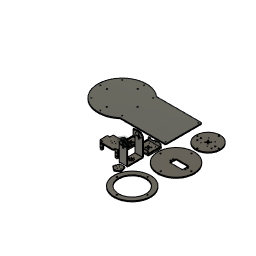
Adaptive Robot (Autodesk Fusion 360 design; units mm, degrees)
Autodesk Fusion 360 part; units mm, degrees
(part 1 of 2)
sketch "Sketch1" plane through (0, 0, 0) normal (0, 0, 1) x (1, 0, 0) in component "Base Plate"
  circle A0 centre (0, 0) radius 80
  line L0 (52.915, 60) -> (52.915, -60)
  line L1 (52.915, -60) -> (199.915, -60)
  line L2 (202.915, -57) -> (202.915, 57)
  line L3 (199.915, 60) -> (52.915, 60)
  line L4 (202.915, 0) -> (52.915, 0) construction
  arc A1 (202.915, 57) -> (199.915, 60) centre (199.915, 57) ccw
  arc A2 (199.915, -60) -> (202.915, -57) centre (199.915, -57) ccw
  circle A3 centre (0, 72) radius 1.5
  line L5 (0, 0) -> (0, 80) construction
  circle A4 centre (-50.9117, 50.9117) radius 1.5
  circle A5 centre (-72, 0) radius 1.5
  circle A6 centre (-50.9117, -50.9117) radius 1.5
  circle A7 centre (0, -72) radius 1.5
  circle A8 centre (50.9117, -50.9117) radius 1.5
  circle A9 centre (50.9117, 50.9117) radius 1.5
  line L6 (-50.9117, 50.9117) -> (50.9117, 50.9117) construction
  line L7 (-50.9117, -50.9117) -> (-50.9117, 50.9117) construction
  circle A10 centre (0, 50.9117) radius 2
  circle A11 centre (-50.9117, 0) radius 2
  circle A12 centre (0, -50.9117) radius 2
  circle A13 centre (50.9117, 0) radius 2
  circle A14 centre (196.915, 54) radius 1.5
  circle A15 centre (196.915, -54) radius 1.5
  point P0 (202.915, 60)
  dimension "d2" = 120
  dimension "d3" = 160
  dimension "d4" = 150
  dimension "d5" = 3
  dimension "d6" = 3
  dimension "d8" = 8
  dimension "d10" = 360
  dimension "d13" = 4
  dimension "d15" = 360
  dimension "d20" = 3
  dimension "d21" = 6
  dimension "d22" = 6
  dimension "d23" = 3
  dimension "d24" = 6
  dimension "d25" = 6
  constraint coincident A0.centre L5.start
  constraint perpendicular L0 L1
  constraint parallel L0 L2
  constraint parallel L1 L3
  constraint coincident A0 L0.end
  constraint vertical L0
  constraint coincident A0 L0.start
  constraint midpoint L0 L4.end
  constraint coincident L2 L4.start
  constraint coincident P0 L2
  constraint coincident P0 L3
  constraint tangent L2 A1
  constraint tangent L3 A1
  constraint tangent L1 A2
  constraint tangent L2 A2
  constraint equal A1 A2
  constraint coincident A0 L5.end
  constraint vertical L5
  constraint coincident A3.centre L5
  constraint coincident A4.centre L6.start
  constraint coincident A9.centre L6.end
  constraint coincident A6.centre L7.start
  constraint midpoint L6 A10.centre
  measures "d2" distance of L1 L3
  measures "d3" diameter of A0
  measures "d4" distance of L0.start P0
  measures "d5" radius of A1
  measures "d6" diameter of A3
  measures "d8" distance of A3.centre L5.end
  measures "d13" diameter of A10
  measures "d20" diameter of A14
  measures "d21" distance of L3 A14.centre
  measures "d22" distance of L2 A14.centre
  measures "d23" diameter of A15
  measures "d24" distance of L1 A15.centre
  measures "d25" distance of L2 A15.centre
extrude "Extrude3" add sketch "Sketch1" along normal blind 3 contours A0 L0 | A0 L1 L2 L3 A1 A2 | A0 L0 | A14 | A15 makes body 1 in component "Base Plate"
extrude "Extrude4" cut sketch "Sketch1" along normal blind 3 contours A14 | A15 bodies 1 in component "Base Plate"
sketch "Sketch1 (2)" plane through (0, 0, 0) normal (0, 0, 1) x (1, 0, 0) in component "CircularL"
  circle A0 centre (131.6018, -175.8664) radius 40
  circle A1 centre (131.6018, -175.8664) radius 4
  circle A2 centre (131.6018, -140.3664) radius 2
  line L0 (131.6018, -175.8664) -> (131.6018, -135.8664) construction
  circle A3 centre (96.1018, -175.8664) radius 2
  circle A4 centre (131.6018, -211.3664) radius 2
  circle A5 centre (167.1018, -175.8664) radius 2
  line L1 (96.1018, -175.8664) -> (167.1018, -175.8664) construction
  circle A6 centre (108.1018, -175.8664) radius 2
  line L2 (108.1018, -175.8664) -> (108.1018, -208.2353) construction
  circle A7 centre (108.1018, -187.8664) radius 2
  circle A8 centre (155.1018, -187.8664) radius 2
  circle A9 centre (155.1018, -175.8664) radius 2
  line L3 (131.6018, -175.8664) -> (159.8861, -147.5821) construction
  circle A10 centre (136.5516, -170.9166) radius 1.5
  circle A11 centre (126.6521, -170.9166) radius 1.5
  circle A12 centre (126.6521, -180.8161) radius 1.5
  circle A13 centre (136.5516, -180.8161) radius 1.5
  line L4 (131.6018, -162.3664) -> (93.9488, -162.3664) construction
  dimension "d30" = 80
  dimension "d31" = 8
  dimension "d32" = 4
  dimension "d33" = 4.5
  dimension "d35" = 360
  dimension "d36" = 4
  dimension "d37" = 12
  dimension "d38" = 4
  dimension "d39" = 12
  dimension "d40" = 45
  dimension "d41" = 3
  dimension "d42" = 7
  dimension "d44" = 360
  dimension "d46" = 13.5
  constraint concentric A0 A1
  constraint coincident A0.centre A1.centre
  constraint coincident A0 L0.end
  constraint vertical L0
  constraint coincident A2.centre L0
  constraint coincident A3.centre L1.start
  constraint coincident A5.centre L1.end
  constraint coincident L1 A6.centre
  constraint coincident A6.centre L2.start
  constraint perpendicular L1 L2
  constraint coincident L2 A7.centre
  constraint coincident A0 L2.end
  constraint symmetric L0 A6 A9
  constraint symmetric L0 A7 A8
  constraint coincident A0 L3.end
  constraint coincident L3 A10.centre
  constraint coincident A0 L4.end
  constraint perpendicular L0 L4
  measures "d30" diameter of A0
  measures "d31" diameter of A1
  measures "d32" diameter of A2
  measures "d33" distance of A2.centre L0.end
  measures "d36" diameter of A6
  measures "d37" distance of A3.centre A6.centre
  measures "d38" diameter of A7
  measures "d39" distance of A6.centre A7.centre
  measures "d40" angle of L1 L3
  measures "d41" diameter of A10
  measures "d42" distance of A0.centre A10.centre
  measures "d46" distance of A0.centre L4.start
extrude "Extrude1" add sketch "Sketch1 (2)" along normal blind 3 separate body makes body 2 in component "CircularL"
sketch "Sketch1 (3)" plane through (0, 0, 0) normal (0, 0, 1) x (1, 0, 0) in component "ServoHolder"
  line L0 (60.9854, -112.0365) -> (103.9854, -112.0365)
  line L1 (103.9854, -112.0365) -> (103.9854, -155.0365)
  line L2 (103.9854, -155.0365) -> (60.9854, -155.0365)
  line L3 (60.9854, -155.0365) -> (60.9854, -112.0365)
  line L4 (82.4854, -112.0365) -> (82.4854, -155.0365) construction
  line L5 (60.9854, -133.5365) -> (103.9854, -133.5365) construction
  circle A0 centre (82.4854, -133.5365) radius 4
  circle A1 centre (95.9854, -123.0365) radius 1
  line L6 (95.9854, -123.0365) -> (95.9854, -155.0365) construction
  circle A2 centre (95.9854, -144.0365) radius 1
  circle A3 centre (68.9854, -144.0365) radius 1
  circle A4 centre (68.9854, -123.0365) radius 1
  dimension "d51" = 43
  dimension "d52" = 43
  dimension "d53" = 8
  dimension "d54" = 2
  dimension "d55" = 11
  dimension "d56" = 8
  constraint horizontal L0
  constraint vertical L1
  constraint horizontal L2
  constraint vertical L3
  constraint midpoint L0 L4.start
  constraint midpoint L2 L4.end
  constraint midpoint L3 L5.start
  constraint midpoint L1 L5.end
  constraint midpoint L5 A0.centre
  constraint coincident A1.centre L6.start
  constraint coincident L2 L6.end
  constraint perpendicular L2 L6
  constraint symmetric L5 A1 A2
  constraint symmetric L4 A1 A4
  constraint symmetric L4 A2 A3
  measures "d51" distance of L1 L3
  measures "d52" distance of L0 L2
  measures "d53" diameter of A0
  measures "d54" diameter of A1
  measures "d55" distance of L0 A1.centre
  measures "d56" distance of L1 A1.centre
extrude "Extrude1'" add sketch "Sketch1 (3)" along normal blind 3 separate body makes body 3 in component "ServoHolder"
sketch "Sketch2" plane through (0, 0, 3) normal (0, 0, 1) x (-1, 0, 0) in component "ServoHolder"
  circle A0 centre (-95.9854, 123.0365) radius 1
  circle A1 centre (-95.9854, 144.0365) radius 1
  circle A2 centre (-68.9854, 123.0365) radius 1
  circle A3 centre (-82.4854, 133.5365) radius 4
  circle A4 centre (-68.9854, 144.0365) radius 1
  line L0 (-60.9854, 155.0365) -> (-103.9854, 155.0365)
  line L1 (-103.9854, 155.0365) -> (-103.9854, 112.0365)
  line L2 (-103.9854, 112.0365) -> (-60.9854, 112.0365)
  line L3 (-60.9854, 112.0365) -> (-60.9854, 155.0365)
  line L4 (-60.9854, 112.0365) -> (-103.9854, 112.0365)
  line L5 (-103.9854, 112.0365) -> (-103.9854, 113.0365)
  line L6 (-103.9854, 113.0365) -> (-60.9854, 113.0365)
  line L7 (-60.9854, 113.0365) -> (-60.9854, 112.0365)
  line L8 (-60.9854, 155.0365) -> (-103.9854, 155.0365)
  line L9 (-103.9854, 155.0365) -> (-103.9854, 154.0365)
  line L10 (-103.9854, 154.0365) -> (-60.9854, 154.0365)
  line L11 (-60.9854, 154.0365) -> (-60.9854, 155.0365)
  dimension "d59" = 1
  dimension "d60" = 1
  constraint horizontal L4
  constraint vertical L5
  constraint horizontal L6
  constraint vertical L7
  constraint coincident L1 L5.end
  constraint coincident L2.end L3.start
  constraint horizontal L8
  constraint vertical L9
  constraint horizontal L10
  constraint vertical L11
  constraint coincident L1 L9.end
  constraint coincident L0.start L3.end
  measures "d59" distance of L0.end L9.end
  measures "d60" distance of L1.end L5.end
extrude "Extrude2" add sketch "Sketch2" along normal blind 3 contours L0 L1 L3 L8 L9 L10 L11 | L1 L2 L3 L4 L5 L6 L7 bodies 3 in component "ServoHolder"
sketch "Sketch3" plane through (0, 0, 3) normal (0, 0, 1) x (-1, 0, 0) in component "ServoHolder"
  line L0 (-60.9854, 154.0365) -> (-103.9854, 154.0365)
  line L1 (-103.9854, 154.0365) -> (-103.9854, 113.0365)
  line L2 (-103.9854, 113.0365) -> (-60.9854, 113.0365)
  line L3 (-60.9854, 113.0365) -> (-60.9854, 154.0365)
  circle A0 centre (-68.9854, 144.0365) radius 1
  circle A1 centre (-82.4854, 133.5365) radius 4
  circle A2 centre (-68.9854, 123.0365) radius 1
  circle A3 centre (-95.9854, 144.0365) radius 1
  circle A4 centre (-95.9854, 123.0365) radius 1
  line L4 (-60.9854, 113.0365) -> (-61.9854, 113.0365)
  line L5 (-61.9854, 113.0365) -> (-61.9854, 154.0365)
  line L6 (-61.9854, 154.0365) -> (-60.9854, 154.0365)
  line L7 (-60.9854, 154.0365) -> (-60.9854, 113.0365)
  line L8 (-103.9854, 113.0365) -> (-102.9854, 113.0365)
  line L9 (-102.9854, 113.0365) -> (-102.9854, 154.0365)
  line L10 (-102.9854, 154.0365) -> (-103.9854, 154.0365)
  line L11 (-103.9854, 154.0365) -> (-103.9854, 113.0365)
  dimension "d63" = 1
  dimension "d64" = 1
  constraint horizontal L4
  constraint vertical L5
  constraint horizontal L6
  constraint vertical L7
  constraint coincident L0 L5.end
  constraint coincident L2.end L3.start
  constraint horizontal L8
  constraint vertical L9
  constraint horizontal L10
  constraint vertical L11
  constraint coincident L0 L9.end
  constraint coincident L1.end L2.start
  measures "d63" distance of L2.end L4.end
  measures "d64" distance of L1.end L8.end
extrude "Extrude3'" add sketch "Sketch3" along normal blind 10 contours L0 L2 L3 L4 L5 L6 L7 | L0 L1 L2 L8 L9 L10 L11 bodies 3 in component "ServoHolder"
sketch "Sketch4" plane through (60.9854, 0, 0) normal (-1, 0, 0) x (0, -1, 0) in component "ServoHolder"
  line L0 (112.0365, 0) -> (155.0365, 0)
  line L1 (155.0365, 0) -> (155.0365, 6)
  line L2 (155.0365, 6) -> (154.0365, 6)
  line L3 (154.0365, 6) -> (154.0365, 13)
  line L4 (154.0365, 13) -> (113.0365, 13)
  line L5 (113.0365, 13) -> (113.0365, 6)
  line L6 (113.0365, 6) -> (112.0365, 6)
  line L7 (112.0365, 6) -> (112.0365, 0)
  line L8 (134.0365, 13) -> (137.5365, 9)
  line L9 (137.5365, 9) -> (141.5365, 9)
  line L10 (141.5365, 9) -> (141.5365, 13)
  line L11 (149.0365, 13) -> (145.5365, 9)
  line L12 (145.5365, 9) -> (141.5365, 9)
  dimension "d67" = 4
  dimension "d68" = 4
  dimension "d69" = 3.5
  dimension "d70" = 21
  constraint coincident L4 L8.start
  constraint horizontal L9
  constraint coincident L4 L10.end
  constraint perpendicular L4 L10
  constraint symmetric L8.start L10 L11.start
  constraint symmetric L8.end L10 L11.end
  constraint symmetric L9.end L10 L12.end
  measures "d67" distance of L8.end L9.end
  measures "d68" distance of L9.end L10.end
  measures "d69" horizontal distance of L8.start L8.end
  measures "d70" distance of L4.end L8.start
extrude "Extrude4'" cut sketch "Sketch4" against normal blind 43 contours L4 L8 L9 L10 | L4 L10 L11 L12 bodies 3 in component "ServoHolder"
sketch "Sketch5" plane through (60.9854, 0, 0) normal (-1, 0, 0) x (0, -1, 0) in component "ServoHolder"
  line L0 (149.0365, 13) -> (145.5365, 9)
  line L1 (145.5365, 9) -> (137.5365, 9)
  line L2 (137.5365, 9) -> (134.0365, 13)
  line L3 (134.0365, 13) -> (113.0365, 13)
  line L4 (113.0365, 13) -> (113.0365, 6)
  line L5 (113.0365, 6) -> (112.0365, 6)
  line L6 (112.0365, 6) -> (112.0365, 0)
  line L7 (112.0365, 0) -> (155.0365, 0)
  line L8 (155.0365, 0) -> (155.0365, 6)
  line L9 (155.0365, 6) -> (154.0365, 6)
  line L10 (154.0365, 6) -> (154.0365, 13)
  line L11 (154.0365, 13) -> (149.0365, 13)
  circle A0 centre (115.5365, 9) radius 1
  circle A1 centre (130.5365, 9) radius 1
  circle A2 centre (151.5365, 9) radius 1
  line L12 (113.0365, 9) -> (154.0365, 9) construction
  dimension "d73" = 2
  dimension "d74" = 2
  dimension "d75" = 2
  dimension "d76" = 4
  dimension "d77" = 2.5
  dimension "d78" = 2.5
  dimension "d79" = 15
  constraint coincident L4 L12.start
  constraint coincident L10 L12.end
  constraint perpendicular L10 L12
  constraint coincident A0.centre L12
  constraint coincident A1.centre L12
  constraint coincident A2.centre L12
  measures "d73" diameter of A0
  measures "d74" diameter of A1
  measures "d75" diameter of A2
  measures "d76" distance of L3 L12
  measures "d77" distance of A2.centre L12.end
  measures "d78" distance of A0.centre L12.start
  measures "d79" distance of A0.centre A1.centre
extrude "Extrude5" cut sketch "Sketch5" against normal blind 43 contours A0 | A1 | A2 bodies 3 in component "ServoHolder"
sketch "Sketch3 (2)" plane through (0, 0, 3) normal (0, 0, 1) x (-1, 0, 0) in component "CircularL"
  circle A0 centre (-136.5516, 170.9166) radius 1.5
  circle A1 centre (-155.1018, 175.8664) radius 2
  circle A2 centre (-155.1018, 187.8664) radius 2
  circle A3 centre (-108.1018, 187.8664) radius 2
  circle A4 centre (-108.1018, 175.8664) radius 2
  circle A5 centre (-167.1018, 175.8664) radius 2
  circle A6 centre (-131.6018, 211.3664) radius 2
  circle A7 centre (-96.1018, 175.8664) radius 2
  circle A8 centre (-131.6018, 140.3664) radius 2
  circle A9 centre (-131.6018, 175.8664) radius 4
  circle A10 centre (-126.6521, 170.9166) radius 1.5
  circle A11 centre (-126.6521, 180.8161) radius 1.5
  circle A12 centre (-136.5516, 180.8161) radius 1.5
  circle A13 centre (-131.6018, 175.8664) radius 40
  circle A14 centre (-359.9097, 287.882) radius 1
  circle A15 centre (-359.9097, 266.882) radius 1
  circle A16 centre (-386.9097, 266.882) radius 1
  circle A17 centre (-386.9097, 287.882) radius 1
extrude "Extrude2'" cut sketch "Sketch3 (2)" against normal blind 3 contours A14 | A15 | A16 | A17 bodies 2 in component "CircularL"
sketch "Sketch6" plane through (0, 0, 3) normal (0, 0, 1) x (-1, 0, 0) in component "ServoHolder"
  line L0 (-102.9854, 154.0365) -> (-102.9854, 113.0365)
  line L1 (-102.9854, 113.0365) -> (-61.9854, 113.0365)
  line L2 (-61.9854, 113.0365) -> (-61.9854, 154.0365)
  line L3 (-61.9854, 154.0365) -> (-102.9854, 154.0365)
  circle A0 centre (-68.9854, 144.0365) radius 1
  circle A1 centre (-82.4854, 133.5365) radius 4
  circle A2 centre (-68.9854, 123.0365) radius 1
  circle A3 centre (-95.9854, 144.0365) radius 1
  circle A4 centre (-95.9854, 123.0365) radius 1
  circle A5 centre (154.3727, 27.0711) radius 1.5
  circle A6 centre (164.2722, 27.0711) radius 1.5
  circle A7 centre (164.2722, 36.9706) radius 1.5
  circle A8 centre (154.3727, 36.9706) radius 1.5
  circle A9 centre (154.3727, 27.0711) radius 1
  circle A10 centre (154.3727, 36.9706) radius 1
  circle A11 centre (164.2722, 27.0711) radius 1
  circle A12 centre (164.2722, 36.9706) radius 1
  dimension "d102" = 2
  dimension "d103" = 2
  dimension "d104" = 2
  dimension "d105" = 2
  constraint concentric A5 A9
  constraint concentric A8 A10
  constraint concentric A6 A11
  constraint concentric A7 A12
  measures "d102" diameter of A9
  measures "d103" diameter of A10
  measures "d104" diameter of A11
  measures "d105" diameter of A12
extrude "Extrude6" cut sketch "Sketch6" against normal blind 3 contours A9 | A10 | A11 | A12 bodies 3 in component "ServoHolder"
sketch "Sketch1 (4)" plane through (0, 0, 0) normal (0, 0, 1) x (1, 0, 0) in component "ServoCutOut"
  circle A0 centre (-2.8865, -157.1678) radius 60
  dimension "d108" = 120
  measures "d108" diameter of A0
extrude "Extrude1''" add sketch "Sketch1 (4)" along normal blind 3 separate body makes body 4 in component "ServoCutOut"
sketch "Sketch2 (2)" plane through (0, 0, 3) normal (0, 0, 1) x (-1, 0, 0) in component "ServoCutOut"
  circle A0 centre (2.8865, 157.1678) radius 60
  circle A1 centre (-196.915, -54) radius 1.5
  circle A2 centre (-196.915, 54) radius 1.5
  circle A3 centre (0, -50.9117) radius 2
  circle A4 centre (-50.9117, -50.9117) radius 1.5
  circle A5 centre (-50.9117, 50.9117) radius 1.5
  circle A6 centre (0, 72) radius 1.5
  circle A7 centre (72, 0) radius 1.5
  circle A8 centre (50.9117, -50.9117) radius 1.5
  circle A9 centre (0, -72) radius 1.5
  circle A10 centre (50.9117, 50.9117) radius 1.5
  circle A11 centre (0, 50.9117) radius 2
  circle A12 centre (50.9117, 0) radius 2
  circle A13 centre (-50.9117, 0) radius 2
  arc A14 (-199.915, 60) -> (-202.915, 57) centre (-199.915, 57) ccw
  line L0 (-199.915, 60) -> (-52.915, 60)
  arc A15 (-52.915, -60) -> (-52.915, 60) centre (0, 0) ccw
  line L1 (-52.915, -60) -> (-199.915, -60)
  arc A16 (-202.915, -57) -> (-199.915, -60) centre (-199.915, -57) ccw
  line L2 (-202.915, -57) -> (-202.915, 57)
extrude "Extrude2''" cut sketch "Sketch2 (2)" against normal blind 3 contours A3 | A11 | A12 | A13 bodies 4 in component "ServoCutOut"
sketch "Sketch3 (3)" plane through (0, 0, 3) normal (0, 0, 1) x (-1, 0, 0) in component "ServoCutOut"
  circle A0 centre (2.8865, 157.1678) radius 60
  line L0 (2.8865, 157.1678) -> (4.4061, 157.1678)
  line L1 (4.4061, 157.1678) -> (62.8865, 157.1678) construction
  line L2 (2.8865, 157.1678) -> (-57.1135, 157.1678) construction
  line L3 (2.8865, 157.1678) -> (2.8865, 155.2869)
  line L4 (2.8865, 155.2869) -> (2.8865, 97.1678) construction
  line L5 (2.8865, 157.1678) -> (2.8865, 217.1678) construction
  line L6 (-28.1135, 167.6678) -> (12.8865, 167.6678)
  line L7 (12.8865, 167.6678) -> (12.8865, 146.6678)
  line L8 (12.8865, 146.6678) -> (-28.1135, 146.6678)
  line L9 (-28.1135, 146.6678) -> (-28.1135, 167.6678)
  line L10 (-28.1135, 167.6678) -> (12.8865, 146.6678) construction
  line L11 (12.8865, 167.6678) -> (-28.1135, 146.6678) construction
  circle A1 centre (12.8865, 157.1678) radius 1.5
  circle A2 centre (-28.1135, 157.1678) radius 1.5
  circle A3 centre (16.8865, 153.1678) radius 2
  circle A4 centre (16.8865, 161.1678) radius 2
  line L12 (-7.6135, 157.1678) -> (-7.6135, 146.6678) construction
  circle A5 centre (-32.1135, 153.1678) radius 2
  circle A6 centre (-32.1135, 161.1678) radius 2
  point P0 (-7.6135, 157.1678)
  point P1 (12.8865, 157.1678)
  dimension "d117" = 41
  dimension "d118" = 21
  dimension "d119" = 10
  dimension "d120" = 3
  dimension "d121" = 3
  dimension "d124" = 4
  dimension "d125" = 4
  dimension "d126" = 4
  constraint coincident A0.centre L0.start
  constraint horizontal L0
  constraint coincident A0 L1.end
  constraint parallel L0 L1
  constraint coincident A0 L2.end
  constraint parallel L0 L2
  constraint perpendicular L0 L3
  constraint coincident A0 L4.end
  constraint perpendicular L0 L4
  constraint coincident A0 L5.end
  constraint perpendicular L1 L5
  constraint horizontal L6
  constraint perpendicular L6 L7
  constraint parallel L6 L8
  constraint parallel L7 L9
  constraint coincident L10 P0
  constraint coincident L11 P0
  constraint coincident L2 P0
  constraint midpoint L7 P1
  constraint coincident P1 A1.centre
  constraint midpoint L9 A2.centre
  constraint symmetric L1 A3 A4
  constraint coincident P0 L12.start
  constraint midpoint L8 L12.end
  constraint symmetric A3 L12 A5
  constraint symmetric A4 L12 A6
  measures "d117" distance of L6.start L6.end
  measures "d118" distance of L6.start L8.end
  measures "d119" distance of A0.centre P1
  measures "d120" diameter of A1
  measures "d121" diameter of A2
  measures "d124" diameter of A3
  measures "d125" distance of L7 A3.centre
  measures "d126" distance of L1 A3.centre
extrude "Extrude4''" cut sketch "Sketch3 (3)" against normal blind 3 contours A3 | A4 | A5 | A6 bodies 4 in component "ServoCutOut"
extrude "Extrude3''" cut sketch "Sketch3 (3)" against normal blind 3 contours L6 L7 L8 L9 A1 A2 | L9 A2 | L9 A2 | L7 A1 | L7 A1 bodies 4 in component "ServoCutOut"
sketch "Sketch1 (5)" plane through (-2.8865, -157.1678, 3) normal (0, 0, 1) x (-1, 0, 0) in component "BearingOutside"
  line L0 (10, 10.5) -> (10, 1.5)
  arc A0 (10, -1.5) -> (10, 1.5) centre (10, 0) ccw
  line L1 (10, -1.5) -> (10, -10.5)
  line L2 (10, -10.5) -> (-31, -10.5)
  line L3 (-31, -10.5) -> (-31, -1.5)
  arc A1 (-31, 1.5) -> (-31, -1.5) centre (-31, 0) ccw
  line L4 (-31, 1.5) -> (-31, 10.5)
  line L5 (-31, 10.5) -> (10, 10.5)
  circle A2 centre (14, 4) radius 2
  circle A3 centre (-35, -4) radius 2
  circle A4 centre (14, -4) radius 2
  circle A5 centre (-35, 4) radius 2
  circle A6 centre (0, 0) radius 60
  circle A7 centre (0, 0) radius 60
  circle A8 centre (0, 0) radius 45
  dimension "d129" = 90
  constraint concentric A6 A7
  constraint concentric A7 A8
  measures "d129" diameter of A8
extrude "Extrude1'''" add sketch "Sketch1 (5)" along normal blind 3 separate body contours A6 A7 makes body 5 in component "BearingOutside"
sketch "Sketch1 (6)" plane through (0, 0, 0) normal (0, 0, 1) x (1, 0, 0) in component "UConnector"
  line L0 (-1.0772, -105.7415) -> (23.9228, -105.7415)
  line L1 (23.9228, -105.7415) -> (23.9228, -160.7415)
  line L2 (23.9228, -160.7415) -> (-1.0772, -160.7415)
  line L3 (-1.0772, -160.7415) -> (-1.0772, -105.7415)
  dimension "d132" = 25
  dimension "d133" = 55
  constraint horizontal L0
  constraint vertical L1
  constraint horizontal L2
  constraint vertical L3
  measures "d132" distance of L0.start L0.end
  measures "d133" distance of L0.end L1.end
extrude "Extrude1''''" add sketch "Sketch1 (6)" along normal blind 3 separate body makes body 6 in component "UConnector"
sketch "Sketch2 (3)" plane through (0, 0, 3) normal (0, 0, 1) x (-1, 0, 0) in component "UConnector"
  line L0 (1.0772, 160.7415) -> (-23.9228, 160.7415)
  line L1 (-23.9228, 160.7415) -> (-23.9228, 105.7415)
  line L2 (-23.9228, 105.7415) -> (1.0772, 105.7415)
  line L3 (1.0772, 105.7415) -> (1.0772, 160.7415)
  line L4 (1.0772, 105.7415) -> (-23.9228, 105.7415)
  line L5 (-23.9228, 105.7415) -> (-23.9228, 108.7415)
  line L6 (-23.9228, 108.7415) -> (1.0772, 108.7415)
  line L7 (1.0772, 108.7415) -> (1.0772, 105.7415)
  line L8 (1.0772, 160.7415) -> (-23.9228, 160.7415)
  line L9 (-23.9228, 160.7415) -> (-23.9228, 157.7415)
  line L10 (-23.9228, 157.7415) -> (1.0772, 157.7415)
  line L11 (1.0772, 157.7415) -> (1.0772, 160.7415)
  dimension "d136" = 3
  dimension "d137" = 3
  constraint horizontal L4
  constraint vertical L5
  constraint horizontal L6
  constraint vertical L7
  constraint coincident L1 L5.end
  constraint coincident L2.end L3.start
  constraint horizontal L8
  constraint vertical L9
  constraint horizontal L10
  constraint vertical L11
  constraint coincident L1 L9.end
  constraint coincident L0.start L3.end
  measures "d136" distance of L0.end L9.end
  measures "d137" distance of L1.end L5.end
extrude "Extrude2'''" add sketch "Sketch2 (3)" along normal blind 65 contours L0 L1 L3 L8 L9 L10 L11 | L1 L2 L3 L4 L5 L6 L7 bodies 6 in component "UConnector"
fillet "Fillet1" radius 12.5 4 edges at (-1.0772, -107.2415, 68) (23.9228, -107.2415, 68) (23.9228, -159.2415, 68) (-1.0772, -159.2415, 68) on bodies 6 in component "UConnector"
sketch "Sketch3 (4)" plane through (0, -160.7415, 0) normal (0, -1, 0) x (1, 0, 0) in component "UConnector"
  arc A0 (23.9228, 55.5) -> (-1.0772, 55.5) centre (11.4228, 55.5) ccw
  line L0 (-1.0772, 55.5) -> (-1.0772, 0)
  line L1 (-1.0772, 0) -> (23.9228, 0)
  line L2 (23.9228, 0) -> (23.9228, 55.5)
  line L3 (-1.0772, 55.5) -> (23.9228, 55.5) construction
  circle A1 centre (11.4228, 55.5) radius 4
  circle A2 centre (4.4228, 55.5) radius 1.5
  circle A3 centre (11.4228, 48.5) radius 1.5
  circle A4 centre (18.4228, 55.5) radius 1.5
  circle A5 centre (11.4228, 62.5) radius 1.5
  dimension "d142" = 8
  dimension "d143" = 3
  dimension "d144" = 7
  dimension "d146" = 360
  constraint coincident A0.end L0.start
  constraint coincident A0.start L2.end
  constraint concentric A0 A1
  constraint coincident L3 A2.centre
  measures "d142" diameter of A1
  measures "d143" diameter of A2
  measures "d144" distance of A0.centre A2.centre
extrude "Extrude3'''" cut sketch "Sketch3 (4)" against normal blind 55 contours A1 | A2 | A3 | A4 | A5 bodies 6 in component "UConnector"
sketch "Sketch4 (2)" plane through (0, 0, 3) normal (0, 0, 1) x (-1, 0, 0) in component "UConnector"
  line L0 (1.0772, 157.7415) -> (-23.9228, 157.7415)
  line L1 (-23.9228, 157.7415) -> (-23.9228, 108.7415)
  line L2 (-23.9228, 108.7415) -> (1.0772, 108.7415)
  line L3 (1.0772, 108.7415) -> (1.0772, 157.7415)
  line L4 (1.0772, 108.7415) -> (-23.9228, 157.7415) construction
  line L5 (-23.9228, 108.7415) -> (1.0772, 157.7415) construction
  circle A0 centre (-11.4228, 133.2415) radius 4
  line L6 (-11.4228, 133.2415) -> (1.0772, 133.2415) construction
  circle A1 centre (-4.4228, 133.2415) radius 1.5
  circle A2 centre (-11.4228, 140.2415) radius 1.5
  circle A3 centre (-18.4228, 133.2415) radius 1.5
  circle A4 centre (-11.4228, 126.2415) radius 1.5
  line L7 (-11.4228, 133.2415) -> (-3.0113, 124.8301) construction
  circle A5 centre (-6.4731, 128.2918) radius 1
  circle A6 centre (-6.4731, 138.1913) radius 1
  circle A7 centre (-16.3726, 138.1913) radius 1
  circle A8 centre (-16.3726, 128.2918) radius 1
  dimension "d149" = 8
  dimension "d150" = 3
  dimension "d151" = 7
  dimension "d153" = 360
  dimension "d154" = 45
  dimension "d155" = 2
  dimension "d156" = 7
  dimension "d158" = 360
  constraint coincident L2.end L3.start
  constraint coincident L0.end L1.start
  constraint coincident L1.end L2.start
  constraint coincident L0.start L3.end
  constraint midpoint L4 A0.centre
  constraint coincident A0.centre L6.start
  constraint midpoint L3 L6.end
  constraint coincident L6 A1.centre
  constraint coincident L7 A5.centre
  measures "d149" diameter of A0
  measures "d150" diameter of A1
  measures "d151" distance of A0.centre A1.centre
  measures "d154" angle of L6 L7
  measures "d155" diameter of A5
  measures "d156" distance of A0.centre A5.centre
extrude "Extrude4'''" cut sketch "Sketch4 (2)" against normal blind 3 contours A0 | A1 | A2 | A3 | A4 | A5 | A6 | A7 | A8 bodies 6 in component "UConnector"
fillet "Fillet2" radius 3 2 edges at (11.4228, -105.7415, 0) (11.4228, -160.7415, 0) on bodies 6 in component "UConnector"
sketch "Sketch1 (7)" plane through (0, 0, 0) normal (0, 0, 1) x (1, 0, 0) in component "SquareUConnector"
  line L0 (-68.0117, -109.9157) -> (-41.0117, -109.9157)
  line L1 (-41.0117, -109.9157) -> (-41.0117, -154.9157)
  line L2 (-41.0117, -154.9157) -> (-68.0117, -154.9157)
  line L3 (-68.0117, -154.9157) -> (-68.0117, -109.9157)
  dimension "d163" = 45
  dimension "d164" = 27
  constraint horizontal L0
  constraint vertical L1
  constraint horizontal L2
  constraint vertical L3
  measures "d163" distance of L0 L2
  measures "d164" distance of L1 L3
extrude "Extrude1'''''" add sketch "Sketch1 (7)" along normal blind 3 separate body makes body 7 in component "SquareUConnector"
sketch "Sketch2 (4)" plane through (0, 0, 3) normal (0, 0, 1) x (-1, 0, 0) in component "SquareUConnector"
  line L0 (68.0117, 154.9157) -> (41.0117, 154.9157)
  line L1 (41.0117, 154.9157) -> (41.0117, 109.9157)
  line L2 (41.0117, 109.9157) -> (68.0117, 109.9157)
  line L3 (68.0117, 109.9157) -> (68.0117, 154.9157)
  line L4 (68.0117, 109.9157) -> (67.0117, 109.9157)
  line L5 (67.0117, 109.9157) -> (67.0117, 154.9157)
  line L6 (67.0117, 154.9157) -> (68.0117, 154.9157)
  line L7 (68.0117, 154.9157) -> (68.0117, 109.9157)
  line L8 (41.0117, 154.9157) -> (42.0117, 154.9157)
  line L9 (42.0117, 154.9157) -> (42.0117, 109.9157)
  line L10 (42.0117, 109.9157) -> (41.0117, 109.9157)
  line L11 (41.0117, 109.9157) -> (41.0117, 154.9157)
  dimension "d167" = 1
  dimension "d168" = 1
  constraint horizontal L4
  constraint vertical L5
  constraint horizontal L6
  constraint vertical L7
  constraint coincident L0 L5.end
  constraint coincident L2.end L3.start
  constraint horizontal L8
  constraint vertical L9
  constraint horizontal L10
  constraint vertical L11
  constraint coincident L2 L9.end
  constraint coincident L0.end L1.start
  measures "d167" distance of L2.end L4.end
  measures "d168" distance of L9.end L1.end
extrude "Extrude2''''" add sketch "Sketch2 (4)" along normal blind 3 contours L0 L2 L3 L4 L5 L6 L7 | L0 L1 L2 L8 L9 L10 L11 bodies 7 in component "SquareUConnector"
sketch "Sketch3 (5)" plane through (0, 0, 3) normal (0, 0, 1) x (-1, 0, 0) in component "SquareUConnector"
  line L0 (42.0117, 154.9157) -> (42.0117, 109.9157)
  line L1 (42.0117, 109.9157) -> (67.0117, 109.9157)
  line L2 (67.0117, 109.9157) -> (67.0117, 154.9157)
  line L3 (67.0117, 154.9157) -> (42.0117, 154.9157)
  line L4 (67.0117, 154.9157) -> (42.0117, 154.9157)
  line L5 (42.0117, 154.9157) -> (42.0117, 151.9157)
  line L6 (42.0117, 151.9157) -> (67.0117, 151.9157)
  line L7 (67.0117, 151.9157) -> (67.0117, 154.9157)
  line L8 (67.0117, 109.9157) -> (42.0117, 109.9157)
  line L9 (42.0117, 109.9157) -> (42.0117, 112.9157)
  line L10 (42.0117, 112.9157) -> (67.0117, 112.9157)
  line L11 (67.0117, 112.9157) -> (67.0117, 109.9157)
  dimension "d171" = 3
  dimension "d172" = 3
  constraint horizontal L4
  constraint vertical L5
  constraint horizontal L6
  constraint vertical L7
  constraint coincident L0 L5.end
  constraint coincident L2.end L3.start
  constraint horizontal L8
  constraint vertical L9
  constraint horizontal L10
  constraint vertical L11
  constraint coincident L0 L9.end
  constraint coincident L1.end L2.start
  measures "d171" distance of L0.start L5.end
  measures "d172" distance of L0.end L9.end
extrude "Extrude3''''" add sketch "Sketch3 (5)" along normal blind 23 contours L0 L2 L3 L4 L5 L6 L7 | L0 L1 L2 L8 L9 L10 L11 bodies 7 in component "SquareUConnector"
fillet "Fillet1'" radius 12.5 2 edges at (-67.0117, -153.4157, 26) (-42.0117, -153.4157, 26) on bodies 7 in component "SquareUConnector"
sketch "Sketch4 (3)" plane through (0, -154.9157, 0) normal (0, -1, 0) x (1, 0, 0) in component "SquareUConnector"
  arc A0 (-42.0117, 13.5) -> (-67.0117, 13.5) centre (-54.5117, 13.5) ccw
  line L0 (-67.0117, 13.5) -> (-67.0117, 6)
  line L1 (-67.0117, 6) -> (-68.0117, 6)
  line L2 (-68.0117, 6) -> (-68.0117, 0)
  line L3 (-68.0117, 0) -> (-41.0117, 0)
  line L4 (-41.0117, 0) -> (-41.0117, 6)
  line L5 (-41.0117, 6) -> (-42.0117, 6)
  line L6 (-42.0117, 6) -> (-42.0117, 13.5)
  line L7 (-67.0117, 13.5) -> (-42.0117, 13.5) construction
  circle A1 centre (-54.5117, 13.5) radius 4
  circle A2 centre (-61.5117, 13.5) radius 1
  circle A3 centre (-54.5117, 6.5) radius 1
  circle A4 centre (-47.5117, 13.5) radius 1
  circle A5 centre (-54.5117, 20.5) radius 1
  dimension "d177" = 8
  dimension "d178" = 2
  dimension "d179" = 7
  dimension "d181" = 360
  constraint coincident A0.end L0.start
  constraint coincident A0.start L6.end
  constraint concentric A0 A1
  constraint coincident L7 A2.centre
  measures "d177" diameter of A1
  measures "d178" diameter of A2
  measures "d179" distance of A0.centre A2.centre
extrude "Extrude5'" cut sketch "Sketch4 (3)" against normal blind 3 contours A2 | A3 | A4 | A5 bodies 7 in component "SquareUConnector"
extrude "Extrude4''''" cut sketch "Sketch4 (3)" against normal blind 45 contours A1 bodies 7 in component "SquareUConnector"
sketch "Sketch5 (2)" plane through (0, -109.9157, 0) normal (0, 1, 0) x (-1, 0, 0) in component "SquareUConnector"
  circle A0 centre (54.5117, 13.5) radius 4
  line L0 (41.0117, 0) -> (68.0117, 0)
  line L1 (68.0117, 0) -> (68.0117, 6)
  line L2 (68.0117, 6) -> (67.0117, 6)
  line L3 (67.0117, 6) -> (67.0117, 26)
  line L4 (67.0117, 26) -> (42.0117, 26)
  line L5 (42.0117, 26) -> (42.0117, 6)
  line L6 (42.0117, 6) -> (41.0117, 6)
  line L7 (41.0117, 6) -> (41.0117, 0)
  circle A1 centre (46.0117, 24) radius 1
  circle A2 centre (54.5117, 6.5) radius 1
  line L8 (54.5117, 6.5) -> (42.0117, 6.5) construction
  line L9 (46.0117, 24) -> (46.0117, 6.5) construction
  circle A3 centre (46.0117, 6.5) radius 1
  line L10 (54.5117, 13.5) -> (54.5117, 17.5) construction
  circle A4 centre (63.0117, 24) radius 1
  circle A5 centre (63.0117, 6.5) radius 1
  dimension "d186" = 2
  dimension "d187" = 4
  dimension "d188" = 2
  dimension "d189" = 2
  constraint coincident A2.centre L8.start
  constraint coincident L5 L8.end
  constraint perpendicular L5 L8
  constraint coincident A1.centre L9.start
  constraint coincident L8 L9.end
  constraint perpendicular L8 L9
  constraint coincident L9.end A3.centre
  constraint coincident A0.centre L10.start
  constraint coincident A0 L10.end
  constraint vertical L10
  constraint symmetric A1 L10 A4
  constraint symmetric A3 L10 A5
  measures "d186" diameter of A1
  measures "d187" distance of L5 A1.centre
  measures "d188" distance of L4 A1.centre
  measures "d189" diameter of A3
extrude "Extrude6'" cut sketch "Sketch5 (2)" against normal blind 3 contours A1 | A3 | A4 | A5 bodies 7 in component "SquareUConnector"
sketch "Sketch6 (2)" plane through (0, 0, 3) normal (0, 0, 1) x (-1, 0, 0) in component "SquareUConnector"
  line L0 (67.0117, 151.9157) -> (42.0117, 151.9157)
  line L1 (42.0117, 151.9157) -> (42.0117, 112.9157)
  line L2 (42.0117, 112.9157) -> (67.0117, 112.9157)
  line L3 (67.0117, 112.9157) -> (67.0117, 151.9157)
  line L4 (67.0117, 112.9157) -> (42.0117, 151.9157) construction
  line L5 (42.0117, 112.9157) -> (67.0117, 151.9157) construction
  circle A0 centre (54.5117, 132.4157) radius 4
  line L6 (54.5117, 132.4157) -> (42.0117, 132.4157) construction
  line L7 (54.5117, 132.4157) -> (42.0117, 119.9157) construction
  dimension "d192" = 8
  dimension "d193" = 45
  constraint coincident L2.end L3.start
  constraint coincident L0.end L1.start
  constraint coincident L1.end L2.start
  constraint coincident L0.start L3.end
  constraint midpoint L4 A0.centre
  constraint coincident A0.centre L6.start
  constraint midpoint L1 L6.end
  constraint coincident L1 L7.end
  measures "d192" diameter of A0
  measures "d193" angle of L6 L7
extrude "Extrude7" cut sketch "Sketch6 (2)" against normal blind 3 contours A0 bodies 7 in component "SquareUConnector"
sketch "Sketch7" plane through (0, 0, 3) normal (0, 0, 1) x (-1, 0, 0) in component "SquareUConnector"
  circle A0 centre (54.5117, 132.4157) radius 4
  line L0 (67.0117, 151.9157) -> (42.0117, 151.9157)
  line L1 (42.0117, 151.9157) -> (42.0117, 112.9157)
  line L2 (42.0117, 112.9157) -> (67.0117, 112.9157)
  line L3 (67.0117, 112.9157) -> (67.0117, 151.9157)
  circle A1 centre (-6.4731, 128.2918) radius 1
  circle A2 centre (-16.3726, 128.2918) radius 1
  circle A3 centre (-6.4731, 138.1913) radius 1
  circle A4 centre (-16.3726, 138.1913) radius 1
extrude "Extrude8" cut sketch "Sketch7" against normal blind 3 contours A1 | A2 | A3 | A4 bodies 7 in component "SquareUConnector"
sketch "Sketch1 (8)" plane through (0, 0, 0) normal (0, 0, 1) x (1, 0, 0) in component "CustomConnection"
  line L0 (-112.7996, -122.7327) -> (-70.7996, -122.7327)
  line L1 (-70.7996, -122.7327) -> (-70.7996, -149.7327)
  line L2 (-70.7996, -149.7327) -> (-112.7996, -149.7327)
  line L3 (-112.7996, -149.7327) -> (-112.7996, -122.7327)
  dimension "d202" = 27
  dimension "d203" = 42
  constraint horizontal L0
  constraint vertical L1
  constraint horizontal L2
  constraint vertical L3
  measures "d202" distance of L0.end L1.end
  measures "d203" distance of L0.start L0.end
extrude "Extrude1''''''" add sketch "Sketch1 (8)" along normal blind 3 separate body makes body 8 in component "CustomConnection"
sketch "Sketch2 (5)" plane through (0, 0, 3) normal (0, 0, 1) x (-1, 0, 0) in component "CustomConnection"
  line L0 (112.7996, 149.7327) -> (70.7996, 149.7327)
  line L1 (70.7996, 149.7327) -> (70.7996, 122.7327)
  line L2 (70.7996, 122.7327) -> (112.7996, 122.7327)
  line L3 (112.7996, 122.7327) -> (112.7996, 149.7327)
  line L4 (112.7996, 122.7327) -> (70.7996, 122.7327)
  line L5 (70.7996, 122.7327) -> (70.7996, 125.7327)
  line L6 (70.7996, 125.7327) -> (112.7996, 125.7327)
  line L7 (112.7996, 125.7327) -> (112.7996, 122.7327)
  dimension "d206" = 3
  constraint horizontal L4
  constraint vertical L5
  constraint horizontal L6
  constraint vertical L7
  constraint coincident L1 L5.end
  constraint coincident L2.end L3.start
  measures "d206" distance of L1.end L5.end
extrude "Extrude2'''''" add sketch "Sketch2 (5)" along normal blind 8 contours L1 L2 L3 L4 L5 L6 L7 bodies 8 in component "CustomConnection"
sketch "Sketch3 (6)" plane through (0, 0, 11) normal (0, 0, 1) x (-1, 0, 0) in component "CustomConnection"
  line L0 (112.7996, 125.7327) -> (70.7996, 125.7327)
  line L1 (70.7996, 125.7327) -> (70.7996, 122.7327)
  line L2 (70.7996, 122.7327) -> (112.7996, 122.7327)
  line L3 (112.7996, 122.7327) -> (112.7996, 125.7327)
  line L4 (91.7996, 122.7327) -> (91.7996, 125.7327) construction
  line L5 (62.7996, 122.7327) -> (120.7996, 122.7327)
  line L6 (120.7996, 122.7327) -> (120.7996, 125.7327)
  line L7 (120.7996, 125.7327) -> (62.7996, 125.7327)
  line L8 (62.7996, 125.7327) -> (62.7996, 122.7327)
  line L9 (62.7996, 122.7327) -> (120.7996, 125.7327) construction
  line L10 (120.7996, 122.7327) -> (62.7996, 125.7327) construction
  point P0 (91.7996, 124.2327)
  dimension "d209" = 58
  dimension "d210" = 3
  constraint midpoint L2 L4.start
  constraint midpoint L0 L4.end
  constraint horizontal L5
  constraint perpendicular L5 L6
  constraint parallel L5 L7
  constraint parallel L6 L8
  constraint coincident L9 P0
  constraint coincident L10 P0
  constraint midpoint L4 P0
  measures "d209" distance of L5.start L5.end
  measures "d210" distance of L5 L7
extrude "Extrude3'''''" add sketch "Sketch3 (6)" along normal blind 24 bodies 8 in component "CustomConnection"
sketch "Sketch4 (4)" plane through (0, -125.7327, 0) normal (0, -1, 0) x (1, 0, 0) in component "CustomConnection"
  line L0 (-112.7996, 3) -> (-70.7996, 3)
  line L1 (-70.7996, 3) -> (-70.7996, 11)
  line L2 (-70.7996, 11) -> (-62.7996, 11)
  line L3 (-62.7996, 11) -> (-62.7996, 35)
  line L4 (-62.7996, 35) -> (-120.7996, 35)
  line L5 (-120.7996, 35) -> (-120.7996, 11)
  line L6 (-120.7996, 11) -> (-112.7996, 11)
  line L7 (-112.7996, 11) -> (-112.7996, 3)
  line L8 (-120.7996, 35) -> (-112.2996, 35)
  line L9 (-112.2996, 35) -> (-112.2996, 32)
  line L10 (-112.2996, 32) -> (-120.7996, 32)
  line L11 (-120.7996, 32) -> (-120.7996, 35)
  line L12 (-91.7996, 35) -> (-91.7996, 26.7547) construction
  line L13 (-71.2996, 32) -> (-62.7996, 32)
  line L14 (-71.2996, 35) -> (-71.2996, 32)
  dimension "d213" = 8.5
  dimension "d214" = 3
  constraint horizontal L8
  constraint vertical L9
  constraint horizontal L10
  constraint vertical L11
  constraint coincident L4.end L5.start
  constraint midpoint L4 L12.start
  constraint perpendicular L4 L12
  constraint symmetric L8.end L12 L14.start
  constraint symmetric L9.end L12 L13.start
  constraint symmetric L10.end L12 L13.end
  measures "d213" distance of L9.end L10.end
  measures "d214" distance of L8.end L9.end
extrude "Extrude4'''''" add sketch "Sketch4 (4)" along normal blind 24 contours L4 L5 L8 L9 L10 L11 | L3 L4 L13 L14 bodies 8 in component "CustomConnection"
fillet "Fillet1''" radius 3 6 edges at (-120.7996, -149.7327, 33.5) (-112.2996, -149.7327, 33.5) (-71.2996, -149.7327, 33.5) (-62.7996, -149.7327, 33.5) (-112.7996, -149.7327, 1.5) (-70.7996, -149.7327, 1.5) on bodies 8 in component "CustomConnection"
sketch "Sketch5 (3)" plane through (0, 0, 35) normal (0, 0, 1) x (-1, 0, 0) in component "CustomConnection"
  arc A0 (65.7996, 149.7327) -> (62.7996, 146.7327) centre (65.7996, 146.7327) ccw
  line L0 (62.7996, 146.7327) -> (62.7996, 122.7327)
  line L1 (62.7996, 122.7327) -> (120.7996, 122.7327)
  line L2 (120.7996, 122.7327) -> (120.7996, 146.7327)
  arc A1 (120.7996, 146.7327) -> (117.7996, 149.7327) centre (117.7996, 146.7327) ccw
  line L3 (117.7996, 149.7327) -> (115.2996, 149.7327)
  arc A2 (115.2996, 149.7327) -> (112.2996, 146.7327) centre (115.2996, 146.7327) ccw
  line L4 (112.2996, 146.7327) -> (112.2996, 125.7327)
  line L5 (112.2996, 125.7327) -> (71.2996, 125.7327)
  line L6 (71.2996, 125.7327) -> (71.2996, 146.7327)
  arc A3 (71.2996, 146.7327) -> (68.2996, 149.7327) centre (68.2996, 146.7327) ccw
  line L7 (68.2996, 149.7327) -> (65.7996, 149.7327)
  line L8 (112.2996, 125.7327) -> (71.2996, 125.7327)
  line L9 (71.2996, 125.7327) -> (71.2996, 122.7327)
  line L10 (71.2996, 122.7327) -> (112.2996, 122.7327)
  line L11 (112.2996, 122.7327) -> (112.2996, 125.7327)
  constraint horizontal L8
  constraint vertical L9
  constraint horizontal L10
  constraint vertical L11
  constraint coincident L1 L9.end
  constraint coincident L4.end L5.start
extrude "Extrude5''" add sketch "Sketch5 (3)" along normal blind 6 contours L1 L5 L8 L9 L10 L11 bodies 8 in component "CustomConnection"
sketch "Sketch6 (3)" plane through (0, 0, 35) normal (0, 0, 1) x (-1, 0, 0) in component "CustomConnection"
  line L0 (112.2996, 125.7327) -> (112.2996, 122.7327)
  line L1 (112.2996, 122.7327) -> (120.7996, 122.7327)
  line L2 (120.7996, 122.7327) -> (120.7996, 146.7327)
  arc A0 (120.7996, 146.7327) -> (117.7996, 149.7327) centre (117.7996, 146.7327) ccw
  line L3 (117.7996, 149.7327) -> (115.2996, 149.7327)
  arc A1 (115.2996, 149.7327) -> (112.2996, 146.7327) centre (115.2996, 146.7327) ccw
  line L4 (112.2996, 146.7327) -> (112.2996, 125.7327)
  circle A2 centre (116.5496, 143.2327) radius 2
  circle A3 centre (116.5496, 133.0327) radius 2
  line L5 (116.5496, 122.7327) -> (116.5496, 123.4086)
  line L6 (116.5496, 123.4086) -> (116.5496, 149.7327) construction
  line L7 (112.2996, 122.7327) -> (112.2996, 125.7327) construction
  line L8 (112.2996, 125.7327) -> (71.2996, 125.7327) construction
  line L9 (71.2996, 125.7327) -> (71.2996, 122.7327) construction
  line L10 (71.2996, 122.7327) -> (112.2996, 122.7327) construction
  line L11 (91.7996, 122.7327) -> (91.7996, 125.7327) construction
  circle A4 centre (67.0496, 133.0327) radius 2
  circle A5 centre (67.0496, 143.2327) radius 2
  dimension "d221" = 4
  dimension "d222" = 4
  dimension "d223" = 6.5
  dimension "d224" = 10.2
  constraint midpoint L1 L5.start
  constraint perpendicular L1 L5
  constraint midpoint L3 L6.end
  constraint perpendicular L3 L6
  constraint coincident A3.centre L6
  constraint coincident A2.centre L6
  constraint midpoint L10 L11.start
  constraint midpoint L8 L11.end
  constraint symmetric A2 L11 A5
  constraint symmetric A3 L11 A4
  measures "d221" diameter of A2
  measures "d222" diameter of A3
  measures "d223" distance of A2.centre L6.end
  measures "d224" distance of A2.centre A3.centre
extrude "Extrude6''" cut sketch "Sketch6 (3)" against normal blind 3 contours A2 | A3 | A4 | A5 bodies 8 in component "CustomConnection"
sketch "Sketch7 (2)" plane through (0, 0, 3) normal (0, 0, 1) x (-1, 0, 0) in component "CustomConnection"
  arc A0 (73.7996, 149.7327) -> (70.7996, 146.7327) centre (73.7996, 146.7327) ccw
  line L0 (70.7996, 146.7327) -> (70.7996, 125.7327)
  line L1 (70.7996, 125.7327) -> (112.7996, 125.7327)
  line L2 (112.7996, 125.7327) -> (112.7996, 146.7327)
  arc A1 (112.7996, 146.7327) -> (109.7996, 149.7327) centre (109.7996, 146.7327) ccw
  line L3 (109.7996, 149.7327) -> (73.7996, 149.7327)
  circle A2 centre (81.4996, 137.7327) radius 1.5
  dimension "d227" = 3
  dimension "d228" = 12
  dimension "d229" = 10.7
  measures "d227" diameter of A2
  measures "d228" distance of L3 A2.centre
  measures "d229" distance of L0 A2.centre
extrude "Extrude7'" cut sketch "Sketch7 (2)" against normal blind 3 contours A2 bodies 8 in component "CustomConnection"
sketch "Sketch1 (9)" plane through (0, 0, 0) normal (0, 0, 1) x (1, 0, 0) in component "Pentagon Connection"
  circle A0 centre (40.978, -203.8778) radius 1
  circle A1 centre (48.0507, -217.6126) radius 1
  line L0 (56.7692, -201.6126) -> (62.1576, -218.1962)
  circle A2 centre (48.0507, -225.6454) radius 1
  line L1 (48.0507, -228.4454) -> (33.9439, -218.1962)
  line L2 (33.9439, -218.1962) -> (39.3322, -201.6126)
  circle A3 centre (59.4946, -217.3309) radius 1
  line L3 (62.1576, -218.1962) -> (48.0507, -228.4454)
  circle A4 centre (56.0507, -213.6126) radius 1
  circle A5 centre (48.0507, -209.6126) radius 1
  circle A6 centre (40.0507, -213.6126) radius 1
  circle A7 centre (36.6068, -217.3309) radius 1
  line L4 (39.3322, -201.6126) -> (56.7692, -201.6126)
  circle A8 centre (55.1234, -203.8778) radius 1
extrude "Extrude1'''''''" add sketch "Sketch1 (9)" along normal blind 3 separate body makes body 9 in component "Pentagon Connection"
sketch "Sketch8" plane through (0, -122.7327, 0) normal (0, 1, 0) x (-1, 0, 0) in component "CustomConnection"
  line L0 (70.7996, 0) -> (112.7996, 0)
  line L1 (112.7996, 0) -> (112.7996, 11)
  line L2 (112.7996, 11) -> (120.7996, 11)
  line L3 (120.7996, 11) -> (120.7996, 35)
  line L4 (120.7996, 35) -> (112.2996, 35)
  line L5 (112.2996, 35) -> (112.2996, 41)
  line L6 (112.2996, 41) -> (71.2996, 41)
  line L7 (71.2996, 41) -> (71.2996, 35)
  line L8 (71.2996, 35) -> (62.7996, 35)
  line L9 (62.7996, 35) -> (62.7996, 11)
  line L10 (62.7996, 11) -> (70.7996, 11)
  line L11 (70.7996, 11) -> (70.7996, 0)
  circle A0 centre (-40.0507, 100.9024) radius 1
  circle A1 centre (-48.0507, 96.9024) radius 1
  circle A2 centre (-48.0507, 104.9024) radius 1
  circle A3 centre (-56.0507, 100.9024) radius 1
extrude "Extrude8'" cut sketch "Sketch8" against normal blind 3 contours A0 | A1 | A2 | A3 bodies 8 in component "CustomConnection"
sketch "Sketch4 (5)" plane through (0, 0, 3) normal (0, 0, 1) x (-1, 0, 0) in component "CircularL"
  circle A0 centre (-108.1018, 175.8664) radius 2
  circle A1 centre (-167.1018, 175.8664) radius 2
  circle A2 centre (-131.6018, 211.3664) radius 2
  circle A3 centre (-96.1018, 175.8664) radius 2
  circle A4 centre (-131.6018, 140.3664) radius 2
  circle A5 centre (-131.6018, 175.8664) radius 4
  circle A6 centre (-126.6521, 180.8161) radius 1.5
  circle A7 centre (-136.5516, 180.8161) radius 1.5
  circle A8 centre (-126.6521, 170.9166) radius 1.5
  circle A9 centre (-136.5516, 170.9166) radius 1.5
  circle A10 centre (-155.1018, 187.8664) radius 2
  circle A11 centre (-155.1018, 175.8664) radius 2
  circle A12 centre (-108.1018, 187.8664) radius 2
  circle A13 centre (-131.6018, 175.8664) radius 40
  line L0 (-131.6018, 175.8664) -> (-131.6018, 176.8421)
  line L1 (-131.6018, 176.8421) -> (-131.6018, 215.8664) construction
  line L2 (-131.6018, 189.3664) -> (-169.2548, 189.3664) construction
  circle A14 centre (-142.1018, 189.3664) radius 1
  line L3 (-131.6018, 175.8664) -> (-135.6018, 175.8664) construction
  circle A15 centre (-121.1018, 189.3664) radius 1
  circle A16 centre (-121.1018, 162.3664) radius 1
  circle A17 centre (-142.1018, 162.3664) radius 1
  dimension "d241" = 13.5
  dimension "d242" = 2
  dimension "d243" = 10.5
  constraint coincident A5.centre A13.centre
  constraint vertical L0
  constraint coincident A13 L1.end
  constraint parallel L0 L1
  constraint coincident L1 L2.start
  constraint coincident A13 L2.end
  constraint perpendicular L1 L2
  constraint coincident L2 A14.centre
  constraint coincident A5 L3.end
  constraint perpendicular L0 L3
  constraint symmetric L1 A14 A15
  constraint symmetric A14 L3 A17
  constraint symmetric L3 A15 A16
  measures "d241" distance of A5.centre L2.start
  measures "d242" diameter of A14
  measures "d243" distance of L2.start A14.centre
extrude "Extrude3''''''" cut sketch "Sketch4 (5)" against normal blind 3 contours A14 | A15 | A16 | A17 bodies 2 in component "CircularL"